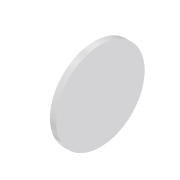
# Autodesk Inventor part: 30_CUBE_openSIM_Beamexpander_Lens_20mm_Edmundoptics
Saved by Autodesk Inventor 2019 (Build 230136000, 136)
## iProperties
Created: 2020-03-03
Part Number: 30_CUBE_openSIM_Beamexpander_Lens_20mm_Edmundoptics
Material: Generic
Document SubType Name: Modeling
Designer: diederichbenedict
Density: 1 g/cm^3
Appearance: Polycarbonate - Clear
Author: diederichbenedict
Autodesk Inventor part; units mm, degrees
ref_plane "YZ Plane" through (0, 0, 0) normal (1, 0, 0) x (0, 1, 0)
ref_plane "XZ Plane" through (0, 0, 0) normal (0, 1, 0) x (-1, 0, 0)
ref_plane "XY Plane" through (0, 0, 0) normal (0, 0, 1) x (1, 0, 0)
sketch "Sketch1" plane through (0, 0, 0) normal (0, 1, 0) x (-1, 0, 0)
  line L0 (0, 0) -> (0, 10)
  line L1 (0, 10) -> (1.4, 10)
  line L2 (0, 0) -> (4.7, 0)
  line L3 (0, 0) -> (4.7, 0) construction
  arc A0 (4.7, 0) -> (1.4, 10) centre (-11.8984, 0.067) ccw
  line L4 (4.7, 0) -> (0, 0)
  line L5 (0, 0) -> (0, 10)
  line L6 (1.4, 10) -> (0, 10)
  dimension "d0" = 10
  dimension "d1" = 1.4
  dimension "d2" = 90
  dimension "d3" = 4.7
  dimension "d4" = 0
  constraints: 14 end point, 3 collinear, 2 horizontal, 2 perpendicular, 2 point on circle, 1 centre point, 1 vertical
  measures "d0" distance of L0.start L0.end
  measures "d1" distance of L0.end L1.end
  measures "d2" angle of L0 L1
  measures "d3" distance of L0.start L2.end
  measures "d4" distance between parallel lines of L2 L3
revolve "Revolution1" add sketch "Sketch1" angle 360 about axis through (0, 0, 0) along (-1, 0, 0)
body "Solid1"
